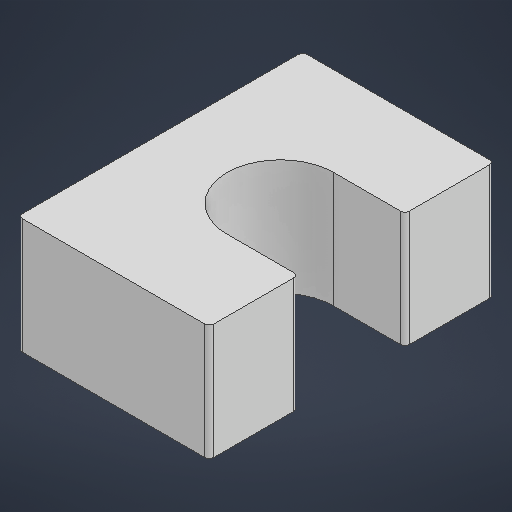
# Autodesk Inventor part: Edge Spacer v2p0
Saved by Autodesk Inventor 2027 (Build 310192060, 192F)
## iProperties
Created: 2026-07-14
Part Number: Edge Spacer v2p0
Material: Generic
Document SubType Name: Modeling
Designer: caleb
Density: 1 g/cm^3
Appearance: Default
Author: caleb
Autodesk Inventor part; units mm, degrees
ref_plane "YZ Plane" through (0, 0, 0) normal (1, 0, 0) x (0, 1, 0)
ref_plane "XZ Plane" through (0, 0, 0) normal (0, 1, 0) x (-1, 0, 0)
ref_plane "XY Plane" through (0, 0, 0) normal (0, 0, 1) x (1, 0, 0)
sketch "Sketch1" plane through (0, 0, 0) normal (0, 1, 0) x (-1, 0, 0)
  line L0 (-2.15, -3.2) -> (2.15, -3.2)
  line L1 (2.15, -3.2) -> (2.15, 3.2)
  line L2 (2.15, 3.2) -> (-2.15, 3.2)
  line L3 (-2.15, 3.2) -> (-2.15, -3.2)
  line L4 (-2.15, -3.2) -> (2.15, 3.2) construction
  line L5 (2.15, -3.2) -> (-2.15, 3.2) construction
  point P0 (0, 0)
  dimension "d0" = 6.4
  dimension "d1" = 4.3
  constraints: 12 end point, 2 midpoint, 2 parallel, 1 horizontal, 1 perpendicular
  measures "d0" distance of L0.end L1.end
  measures "d1" distance of L1.end L2.end
extrude "Extrusion1" add sketch "Sketch1" along normal blind 2.6
sketch "Sketch2" plane through (0, 2.6, 0) normal (0, 1, 0) x (1, 0, 0)
  line L0 (2.15, -3.2) -> (2.15, 3.2) projected
  line L1 (2.15, -1.2) -> (0.55, -1.2)
  line L2 (2.15, 1.2) -> (0.55, 1.2)
  arc A0 (0.55, 1.2) -> (0.55, -1.2) centre (0.55, 0) ccw
  point P0 (0, 0)
  dimension "d4" = 2.4
  dimension "d5" = 1.2
  dimension "d6" = 1.6
  dimension "d7" = 1.2
  constraints: 4 end point, 2 perpendicular, 2 point on circle, 2 point on line, 1 centre point, 1 vertical alignment
  measures "d4" distance between parallel lines of L1 L2
  measures "d5" distance from line of L1 point (0, 0)
  measures "d6" distance of L1.start L1.end
  measures "d7" radius of A0
extrude "Extrusion2" cut sketch "Sketch2" against normal through all
fillet "Fillet1" radius 0.1 6 edges at (2.15, 1.3, 3.2) (-2.15, 1.3, 3.2) (-2.15, 1.3, -3.2) (2.15, 1.3, -3.2) (2.15, 1.3, -1.2) (2.15, 1.3, 1.2)
equation "\"d5\" = 0.5 * d4"
body "Solid1"
